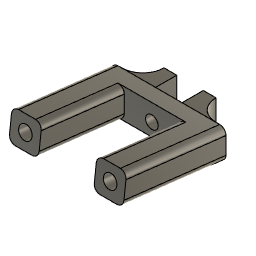
Angled Carbon Components Holder v3 (Autodesk Fusion 360 design; units mm, degrees)
Autodesk Fusion 360 part; units mm, degrees
note: some values were not read from the file. Set by a fixed rule: which face or edge a step refers to.
sketch "Sketch1" plane through (0, 0, 0) normal (0, 1, 0) x (1, 0, 0)
  circle A0 centre (0, 0) radius 1.5
  line L0 (0, 0) -> (10, 0)
  line L1 (0, 1.5) -> (0, -1.5)
  line L2 (-13.5, -3.5) -> (13.5, -3.5)
  line L3 (13.5, -3.5) -> (13.5, 3.5)
  line L4 (13.5, 3.5) -> (-13.5, 3.5)
  line L5 (-13.5, 3.5) -> (-13.5, -3.5)
  line L6 (-13.5, -3.5) -> (13.5, 3.5) construction
  line L7 (13.5, -3.5) -> (-13.5, 3.5) construction
  line L8 (0, 3.5) -> (0, -3.5)
  dimension "d1" = 3
  dimension "d2" = 10
  dimension "d10" = 27
  dimension "d11" = 7
  constraint coincident A0.centre L0.start
  constraint horizontal L0
  constraint coincident A0 L1.start
  constraint coincident A0 L1.end
  constraint perpendicular L0 L1
  constraint horizontal L2
  constraint perpendicular L2 L3
  constraint parallel L2 L4
  constraint parallel L3 L5
  constraint coincident L6 A0.centre
  constraint coincident L7 A0.centre
  constraint midpoint L4 L8.start
  constraint midpoint L2 L8.end
  measures "d1" diameter of A0
  measures "d2" distance of A0.centre L0.end
  measures "d10" distance of L3.end L4.end
  measures "d11" distance of L2.end L3.end
ref_plane "WorkPlane1" through (5, 0, 0) normal (0, -0.993171, 0.116671) x (1, 0, 0)
sketch "Sketch2" plane through (5, 0, 0) normal (0, -0.993171, 0.116671) x (1, 0, 0)
  circle A0 centre (5, 0) radius 1.6
  line L0 (1.5, 3.5) -> (8.5, 3.5)
  line L1 (8.5, 3.5) -> (8.5, -3.5)
  line L2 (8.5, -3.5) -> (1.5, -3.5)
  line L3 (1.5, -3.5) -> (1.5, 3.5)
  line L4 (1.5, 3.5) -> (8.5, -3.5) construction
  line L5 (8.5, 3.5) -> (1.5, -3.5) construction
  point P0 (5, 0)
  point P1 (5, 0)
  dimension "d5" = 3.2
  dimension "d8" = 7
  dimension "d9" = 7
  constraint coincident P0 A0.centre
  constraint horizontal L0
  constraint perpendicular L0 L1
  constraint parallel L0 L2
  constraint parallel L1 L3
  constraint coincident L4 P1
  constraint coincident L5 P1
  measures "d5" diameter of A0
  measures "d8" distance of L1.end L2.end
  measures "d9" distance of L0.end L1.end
extrude "Extrude1" add sketch "Sketch1" against normal blind 4 contours A0 L2 L3 L4 L8
extrude "Extrude2" add sketch "Sketch2" along normal blind 20
sketch "Sketch6" plane through (0, 0, 0) normal (-1, 0, 0) x (0, -1, 0)
  line L0 (0, 3.5) -> (0, 1.5)
  line L1 (0, 1.5) -> (4, 1.5)
  line L2 (4, 1.5) -> (4, 3.5)
  line L3 (4, 3.5) -> (0, 3.5)
  line L4 (0, 3.5) -> (-1.2912, 3.5)
  line L5 (-1.2912, 3.5) -> (-1.2912, -0.2888)
  line L6 (-1.2912, -0.2888) -> (0, -0.2888)
  line L7 (0, -0.2888) -> (0, 3.5)
  constraint horizontal L4
  constraint vertical L5
  constraint horizontal L6
  constraint vertical L7
  constraint coincident L0.start L3.end
extrude "Extrude9" cut sketch "Sketch6" against normal blind 21 contours L0 L4 L5 L6 L7
extrude "Extrude10" cut 1 faces at (11.1667, 0.1366, 3.5) along direction (0, 0, 1) blind 3
extrude "Extrude3" add 1 faces at (9.9601, -20.1977, -0.5122) along direction (0, -0.993171, 0.116671) blind 4
mirror "Mirror1" about plane through (0, 0, 1.5) normal (-1, 0, 0) of bodies 1 merged
extrude "Extrude4" cut 1 faces at (4.5, -1.3333, -3.5) along direction (0, 0, 1) blind 0.5
extrude "Extrude5" add 2 faces at (-11.1667, -4, -3.0361) (8.8333, -4, -3.0361) along direction (0, 1, 0) blind 4
sketch "Sketch3" plane through (6.5, 0, 0) normal (-1, 0, 0) x (0, -1, 0)
  line L0 (0, 3.5) -> (4, 3.5)
  line L1 (4, 3.5) -> (4, -3)
  line L2 (4, -3) -> (0, -3)
  line L3 (0, 3.5241) -> (0, 3.5)
  line L4 (0, -3.0542) -> (4, -3.0542)
  line L5 (4, -3.0542) -> (24.2444, -0.676)
  line L6 (24.2444, -0.676) -> (23.4277, 6.2762)
  line L7 (23.4277, 6.2762) -> (0, 3.5241)
  line L8 (4, -3.0542) -> (4, -3)
  line L9 (0, -3) -> (0, -3.0542)
  constraint coincident L4.end L5.start
  constraint coincident L1.end L2.start
extrude "Extrude6" add sketch "Sketch3" along normal blind 13 contours L2 L4 L8 L9
sketch "Sketch4" plane through (6.5, 0, 0) normal (-1, 0, 0) x (0, -1, 0)
  line L0 (4, 3.5) -> (4, -3.0542)
  line L1 (4, -3.0542) -> (24.2444, -0.676)
  line L2 (24.2444, -0.676) -> (23.4277, 6.2762)
  line L3 (23.4277, 6.2762) -> (0, 3.5241)
  line L4 (0, 3.5) -> (4, 3.5)
  line L5 (4, 3.5) -> (4, 3.994)
  line L6 (0, 3.5241) -> (0, 3.5)
  constraint coincident L0.start L4.end
  constraint coincident L3 L5.end
  constraint perpendicular L4 L5
extrude "Extrude7" add sketch "Sketch4" along normal blind 13 contours L3 L4 L5 L6
sketch "Sketch5" plane through (13.5, 0, 0) normal (1, 0, 0) x (0, 1, 0)
  line L0 (0, -3.0542) -> (0, 3.5241)
  line L1 (-23.4277, 6.2762) -> (-24.2444, -0.676)
  line L2 (0, 3.5241) -> (0.6416, 3.5241)
  line L3 (0.6416, 3.5241) -> (0.6416, 1.7327)
  line L4 (0.6416, 1.7327) -> (0, 1.7327)
  line L5 (0, 1.7327) -> (0, 3.5241)
  line L6 (-4, -3.0542) -> (0, -3.0542)
  line L7 (0, 3.5241) -> (-23.4277, 6.2762)
  line L8 (-24.2444, -0.676) -> (-4, -3.0542)
  constraint horizontal L2
  constraint vertical L3
  constraint horizontal L4
  constraint vertical L5
  constraint coincident L0.end L2.start
fillet "Fillet3" radius 1.5 8 edges at (-13.5, -11.7139, 4.9001) (13.5, -11.7139, 4.9001) (6.5, -13.7139, 5.1351) (-6.5, -13.7139, 5.1351) (6.5, -14.1222, -1.8651) (13.5, -14.1222, -1.8651) (-6.5, -14.1222, -1.8651) (-13.5, -14.1222, -1.8651)
sketch "Sketch7" plane through (0, 0, 0) normal (0, 1, 0) x (-1, 0, 0)
  circle A0 centre (0, 0) radius 1.5
  ellipse E0 centre (12, -2.0138) end of major axis (12, -3.5241) minor radius 1.5 (13.0873, -3.0542) -> (13.5, -2.0138) ccw
  line L0 (13.5, -2.0138) -> (13.5, 2.0138)
  ellipse E1 centre (12, 2.0138) end of major axis (12, 3.5241) minor radius 1.5 (13.5, 2.0138) -> (12, 3.5241) ccw
  line L1 (12, 3.5241) -> (-12, 3.5241)
  ellipse E2 centre (-12, 2.0138) end of major axis (-12, 3.5241) minor radius 1.5 (-12, 3.5241) -> (-13.5, 2.0138) ccw
  line L2 (-13.5, 2.0138) -> (-13.5, -2.0138)
  ellipse E3 centre (-12, -2.0138) end of major axis (-12, -3.5241) minor radius 1.5 (-13.5, -2.0138) -> (-13.0873, -3.0542) ccw
  line L3 (-13.0873, -3.0542) -> (13.0873, -3.0542)
  line L4 (3.125, 3.0625) -> (-3.125, 3.0625)
  line L5 (-3.125, 3.0625) -> (-3.125, -3.0625)
  line L6 (-3.125, -3.0625) -> (3.125, -3.0625)
  line L7 (3.125, -3.0625) -> (3.125, 3.0625)
  line L8 (3.125, 3.0625) -> (-3.125, -3.0625) construction
  line L9 (-3.125, 3.0625) -> (3.125, -3.0625) construction
  line L10 (-3.125, 3.0625) -> (-3.125, 3.5241)
  line L11 (3.125, 3.0625) -> (3.125, 3.5241)
  line L12 (3.125, 3.5241) -> (6.125, 3.5241)
  line L13 (6.125, 3.5241) -> (6.125, -3.0542)
  line L14 (6.125, -3.0542) -> (3.125, -3.0542)
  line L15 (3.125, -3.0542) -> (3.125, 3.5241)
  line L16 (-3.125, 3.5241) -> (-6.125, 3.5241)
  line L17 (-6.125, 3.5241) -> (-6.125, -3.0542)
  line L18 (-6.125, -3.0542) -> (-3.125, -3.0542)
  line L19 (-3.125, -3.0542) -> (-3.125, 3.5241)
  dimension "d40" = 6.25
  dimension "d41" = 6.125
  dimension "d42" = 3
  dimension "d43" = 3
  constraint horizontal L4
  constraint perpendicular L4 L5
  constraint parallel L4 L6
  constraint parallel L5 L7
  constraint coincident L8 A0.centre
  constraint coincident L9 A0.centre
  constraint coincident A0.centre origin
  constraint coincident L1 L10.end
  constraint perpendicular L1 L10
  constraint coincident L1 L11.end
  constraint perpendicular L1 L11
  constraint horizontal L12
  constraint vertical L13
  constraint horizontal L14
  constraint vertical L15
  constraint horizontal L16
  constraint vertical L17
  constraint horizontal L18
  constraint vertical L19
  measures "d40" distance of L5.end L6.end
  measures "d41" distance of L4.end L5.end
  measures "d42" distance of L11.end L12.end
  measures "d43" distance of L10.end L16.end
extrude "Extrude11" add sketch "Sketch7" along normal blind 5 contours L1 L3 L7 L11 L12 L13 L14 L15 | L1 L3 L5 L10 L16 L17 L18 L19
fillet "Fillet4" radius 5 2 edges at (-6.125, 0, 0.2349) (6.125, 0, 0.2349)
